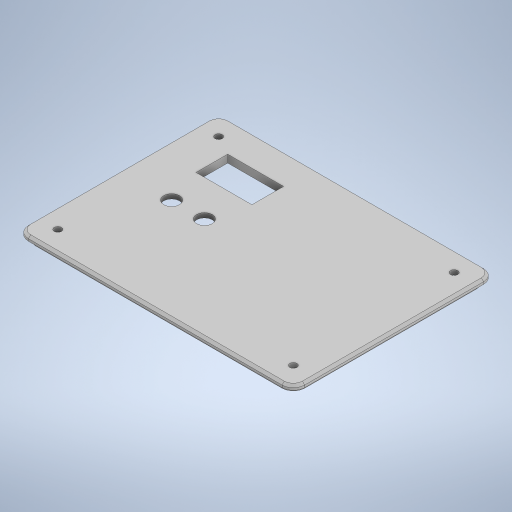
# Autodesk Inventor part: housing_top_v_2
Saved by Autodesk Inventor 2023 (Build 270158000, 158)
## iProperties
Created: 2023-10-04
Part Number: housing_top_v_2
Material: Generic
Document SubType Name: Modeling
Designer: mark
Density: 1 g/cm^3
Appearance: Default
Author: mark
Autodesk Inventor part; units mm, degrees
ref_plane "YZ Plane" through (0, 0, 0) normal (1, 0, 0) x (0, 1, 0)
ref_plane "XZ Plane" through (0, 0, 0) normal (0, 1, 0) x (-1, 0, 0)
ref_plane "XY Plane" through (0, 0, 0) normal (0, 0, 1) x (1, 0, 0)
sketch "Sketch1" plane through (0, 0, 0) normal (0, 1, 0) x (-1, 0, 0)
  line L0 (66.5812, -42.2738) -> (-55.4188, -42.2738)
  line L1 (-55.4188, -42.2738) -> (-55.4188, 46.7262)
  line L2 (-55.4188, 46.7262) -> (66.5812, 46.7262)
  line L3 (66.5812, 46.7262) -> (66.5812, -42.2738)
  point P0 (0, 0)
  dimension "d0" = 122
  dimension "d1" = 89
  constraints: 8 end point, 2 parallel, 1 horizontal, 1 perpendicular
  measures "d0" distance of L1.end L2.end
  measures "d1" distance of L0.end L1.end
extrude "Extrusion1" add sketch "Sketch1" along normal blind 2
sketch "Sketch2" plane through (0, 0, 0) normal (0, -1, 0) x (1, 0, 0)
  line L0 (53.8188, -40.6738) -> (-64.9812, -40.6738)
  line L1 (-64.9812, -40.6738) -> (-64.9812, 45.1262)
  line L2 (-64.9812, 45.1262) -> (53.8188, 45.1262)
  line L3 (53.8188, 45.1262) -> (53.8188, -40.6738)
  line L4 (55.4188, -42.2738) -> (-66.5812, -42.2738) projected
  line L5 (55.4188, 46.7262) -> (55.4188, -42.2738) projected
  line L6 (-66.5812, 46.7262) -> (55.4188, 46.7262) projected
  line L7 (-66.5812, -42.2738) -> (-66.5812, 46.7262) projected
  line L8 (52.4188, -39.2738) -> (-63.5812, -39.2738)
  line L9 (-63.5812, -39.2738) -> (-63.5812, 43.7262)
  line L10 (-63.5812, 43.7262) -> (52.4188, 43.7262)
  line L11 (52.4188, 43.7262) -> (52.4188, -39.2738)
  point P0 (0, 0)
  dimension "d4" = 1.6
  dimension "d5" = 1.6
  dimension "d6" = 1.6
  dimension "d7" = 1.6
  dimension "d8" = 1.4
  dimension "d9" = 1.4
  dimension "d10" = 1.4
  dimension "d11" = 1.4
  constraints: 16 end point, 4 parallel, 2 horizontal, 2 perpendicular
  measures "d4" distance between parallel lines of L4 L0
  measures "d5" distance between parallel lines of L5 L3
  measures "d6" distance between parallel lines of L6 L2
  measures "d7" distance between parallel lines of L7 L1
  measures "d8" distance between parallel lines of L0 L8
  measures "d9" distance between parallel lines of L3 L11
  measures "d10" distance between parallel lines of L2 L10
  measures "d11" distance between parallel lines of L1 L9
extrude "Extrusion2" add sketch "Sketch2" along normal blind 1.8 contours L0 L1 L2 L3
sketch "Sketch3" plane through (0, 2, 0) normal (0, 1, 0) x (1, 0, 0)
  line L0 (55.4188, 42.2738) -> (-66.5812, 42.2738) projected
  line L1 (-66.5812, 42.2738) -> (-66.5812, -46.7262) projected
  point P0 (0, 0)
  point P1 (-57.5812, 33.2738)
  dimension "d14" = 9
  dimension "d15" = 9
  measures "d14" distance from line of L0 point (-57.581, 33.274)
  measures "d15" distance from line of L1 point (-57.581, 33.274)
hole "Hole1" at (-57.5812, 2, -33.2738) direction (0, -1, 0) diameter 3.2 end through all
pattern_linear "Rectangular Pattern1" count 2 spacing 71 along (0, 0, 1) count 2 spacing 104 along (1, 0, 0) of "Hole1"
fillet "Fillet1" radius 5 12 edges at (-66.5812, 1, 46.7262) (-64.9812, -0.9, 45.1262) (-63.5812, -0.9, 43.7262) (-66.5812, 1, -42.2738) (-64.9812, -0.9, -40.6738) (-63.5812, -0.9, -39.2738) (55.4188, 1, -42.2738) (53.8188, -0.9, -40.6738) (52.4188, -0.9, -39.2738) (52.4188, -0.9, 43.7262) (53.8188, -0.9, 45.1262) (55.4188, 1, 46.7262)
chamfer "Chamfer1" distance 1 angle 45 8 edges at (-5.5812, 2, -42.2738) (-65.1167, 2, -40.8093) (-66.5812, 2, 2.2262) (-65.1167, 2, 45.2618) (-5.5812, 2, 46.7262) (53.9543, 2, 45.2618) (55.4188, 2, 2.2262) (53.9543, 2, -40.8093)
sketch "Sketch4" plane through (0, 2, 0) normal (0, 1, 0) x (1, 0, 0)
  line L0 (-48.8812, 28.5738) -> (-24.1812, 28.5738)
  line L1 (-24.1812, 28.5738) -> (-24.1812, 14.5738)
  line L2 (-24.1812, 14.5738) -> (-48.8812, 14.5738)
  line L3 (-48.8812, 14.5738) -> (-48.8812, 28.5738)
  line L4 (50.4188, 42.2738) -> (-61.5812, 42.2738) projected
  line L5 (-66.5812, 37.2738) -> (-66.5812, -41.7262) projected
  circle A0 centre (-43.6812, -1.3962) radius 3.5
  circle A1 centre (-29.1812, -1.3962) radius 3.5
  point P0 (0, 0)
  dimension "d33" = 24.7
  dimension "d34" = 14
  dimension "d35" = 13.7
  dimension "d36" = 17.7
  dimension "d37" = 7
  dimension "d38" = 7
  dimension "d39" = 22.9
  dimension "d40" = 14.5
  dimension "d41" = 43.67
  dimension "d42" = 43.67
  constraints: 8 end point, 2 centre point, 2 parallel, 1 horizontal, 1 perpendicular
  measures "d33" distance of L1.end L2.end
  measures "d34" distance of L0.end L1.end
  measures "d35" distance between parallel lines of L4 L0
  measures "d36" distance between parallel lines of L5 L3
  measures "d37" diameter of A0
  measures "d38" diameter of A1
  measures "d39" distance from line of L5 A0.centre
  measures "d40" distance of A0.centre A1.centre
  measures "d41" distance from line of L4 A1.centre
  measures "d42" distance from line of L4 A0.centre
extrude "Extrusion3" cut sketch "Sketch4" against normal through all
sketch "Sketch5" plane through (0, 0, 0) normal (0, -1, 0) x (1, 0, 0)
  line L0 (-48.8812, -14.5738) -> (-24.1812, -14.5738) projected
  line L1 (-48.8812, -14.5738) -> (-24.1812, -14.5738)
  line L2 (-24.1812, -14.5738) -> (-24.1812, -28.5738)
  line L3 (-24.1812, -28.5738) -> (-48.8812, -28.5738)
  line L4 (-48.8812, -28.5738) -> (-48.8812, -14.5738)
  line L5 (-49.8812, -13.5738) -> (-23.1812, -13.5738)
  line L6 (-23.1812, -13.5738) -> (-23.1812, -29.5738)
  line L7 (-23.1812, -29.5738) -> (-49.8812, -29.5738)
  line L8 (-49.8812, -29.5738) -> (-49.8812, -13.5738)
  point P0 (0, 0)
  dimension "d45" = 1
  dimension "d46" = 1
  dimension "d47" = 1
  dimension "d48" = 1
  constraints: 16 end point, 4 parallel, 2 horizontal, 2 perpendicular
  measures "d45" distance between parallel lines of L0 L5
  measures "d46" distance between parallel lines of L4 L8
  measures "d47" distance between parallel lines of L7 L3
  measures "d48" distance between parallel lines of L6 L2
extrude "Extrusion4" add sketch "Sketch5" along normal blind 1.4
equation "\"d5\" = d4"
equation "\"d6\" = d4"
equation "\"d7\" = d4"
equation "\"d9\" = d8"
equation "\"d10\" = d8"
equation "\"d11\" = d8"
equation "\"d42\" = d41"
equation "\"d46\" = d45"
equation "\"d47\" = d45"
equation "\"d48\" = d45"
body "Solid1"
